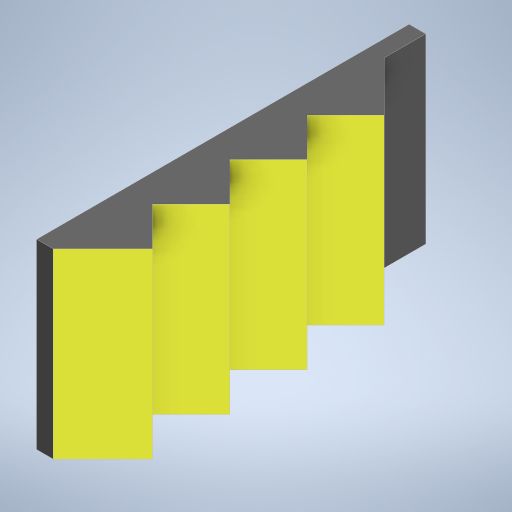
# Autodesk Inventor part: finger
Saved by Autodesk Inventor 2024.1 (Build 281209000, 209)
## iProperties
Created: 2025-01-27
Part Number: finger
Material: 一般
Document SubType Name: Modeling
Designer: hibik
Density: 1 g/cm^3
Appearance: 既定
Author: hibik
Autodesk Inventor part; units mm, degrees
ref_plane "YZ Plane" through (0, 0, 0) normal (1, 0, 0) x (0, 1, 0)
ref_plane "XZ Plane" through (0, 0, 0) normal (0, 1, 0) x (-1, 0, 0)
ref_plane "XY Plane" through (0, 0, 0) normal (0, 0, 1) x (1, 0, 0)
sketch "スケッチ1" plane through (0, 0, 0) normal (1, 0, 0) x (0, 1, 0)
  line L0 (0, 0) -> (22, 0)
  line L1 (22, 0) -> (22, 45)
  line L2 (22, 45) -> (0, 45)
  line L3 (0, 45) -> (0, 0)
  dimension "d0" = 22
  dimension "d1" = 45
  constraints: 8 end point, 2 parallel, 1 horizontal, 1 perpendicular
  measures "d0" distance of L0.start L0.end
  measures "d1" distance of L0.end L1.end
extrude "押し出し1" add sketch "スケッチ1" along normal blind 2
sketch "スケッチ2" plane through (0, 22, 45) normal (0, 1, 0) x (1, 0, 0)
  line L0 (0, 0) -> (2, 0) projected
  line L1 (2, 0) -> (8, 6)
  line L2 (8, 6) -> (3.3333, 10.6667)
  line L3 (3.3333, 10.6667) -> (8, 15.3333)
  line L4 (8, 15.3333) -> (3.3333, 20)
  line L5 (3.3333, 20) -> (8, 24.6667)
  line L6 (8, 24.6667) -> (3.3333, 29.3333)
  line L7 (3.3333, 29.3333) -> (8, 34)
  line L8 (8, 34) -> (2, 40)
  line L9 (2, 45) -> (2, 0) projected
  point P0 (0, 45)
  dimension "d4" = 40
  dimension "d5" = 6
  constraints: 16 end point, 8 perpendicular, 5 parallel, 1 point on line
  measures "d4" distance of L0.end L8.end
  measures "d5" distance from line of L9 L1.end
extrude "押し出し2" add sketch "スケッチ2" against normal up to surface (22 mm away)
